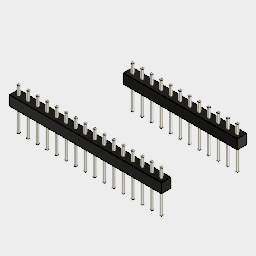
Standard Feather Pins (Autodesk Fusion 360 design; units mm, degrees)
Autodesk Fusion 360 part; units mm, degrees
note: some values were not read from the file. Chosen so that the rebuilt part matches the saved one: which bodies a step acts on.
sketch "pcb" plane through (0, 0, 0) normal (0, 0, 1) x (1, 0, 0)
  line L0 (0, 0) -> (51.2, 0)
  line L1 (51.2, 0) -> (51.2, 22.8)
  line L2 (51.2, 22.8) -> (0, 22.8)
  line L3 (0, 22.8) -> (0, 0)
  circle A0 centre (2.54, 2.54) radius 1.25
  circle A1 centre (2.54, 20.32) radius 1.25
  circle A2 centre (48.26, 20.32) radius 1.25
  circle A3 centre (48.26, 2.54) radius 1.25
  line L4 (0, 11.4) -> (51.2, 11.4) construction
  line L5 (25.6, 22.8) -> (25.6, 0) construction
  line L6 (0, 1.27) -> (51.2, 1.27) construction
  circle A4 centre (24.33, 1.27) radius 0.35
  circle A5 centre (21.79, 1.27) radius 0.35
  circle A6 centre (19.25, 1.27) radius 0.35
  circle A7 centre (16.71, 1.27) radius 0.35
  circle A8 centre (14.17, 1.27) radius 0.35
  circle A9 centre (11.63, 1.27) radius 0.35
  circle A10 centre (6.55, 1.27) radius 0.35
  circle A11 centre (26.87, 1.27) radius 0.35
  circle A12 centre (29.41, 1.27) radius 0.35
  circle A13 centre (31.95, 1.27) radius 0.35
  circle A14 centre (34.49, 1.27) radius 0.35
  circle A15 centre (39.57, 1.27) radius 0.35
  circle A16 centre (37.03, 1.27) radius 0.35
  circle A17 centre (42.11, 1.27) radius 0.35
  circle A18 centre (44.65, 1.27) radius 0.35
  circle A19 centre (44.65, 21.53) radius 0.35
  circle A20 centre (39.57, 21.53) radius 0.35
  circle A21 centre (34.49, 21.53) radius 0.35
  circle A22 centre (31.95, 21.53) radius 0.35
  circle A23 centre (29.41, 21.53) radius 0.35
  circle A24 centre (26.87, 21.53) radius 0.35
  circle A25 centre (42.11, 21.53) radius 0.35
  circle A26 centre (37.03, 21.53) radius 0.35
  circle A27 centre (24.33, 21.53) radius 0.35
  circle A28 centre (21.79, 21.53) radius 0.35
  circle A29 centre (19.25, 21.53) radius 0.35
  circle A30 centre (16.71, 21.53) radius 0.35
  line L7 (0, 2.54) -> (51.2, 2.54) construction
  circle A31 centre (9.09, 1.27) radius 0.35
  line L8 (45.92, 2.54) -> (5.28, 2.54)
  line L9 (5.28, 2.54) -> (5.28, 0)
  line L10 (5.28, 0) -> (45.92, 0)
  line L11 (45.92, 0) -> (45.92, 2.54)
  line L12 (45.92, 2.54) -> (5.28, 0) construction
  line L13 (5.28, 2.54) -> (45.92, 0) construction
  line L14 (45.92, 22.8) -> (15.44, 22.8)
  line L15 (15.44, 22.8) -> (15.44, 20.26)
  line L16 (15.44, 20.26) -> (45.92, 20.26)
  line L17 (45.92, 20.26) -> (45.92, 22.8)
  line L18 (45.92, 22.8) -> (15.44, 20.26) construction
  line L19 (15.44, 22.8) -> (45.92, 20.26) construction
  point P0 (25.6, 1.27)
  point P1 (30.68, 21.53)
  dimension "d1" = 51.2
  dimension "d2" = 22.8
  dimension "d3" = 2.5
  dimension "d4" = 2.54
  dimension "d5" = 2.54
  dimension "d6" = 2.5
  dimension "d7" = 2.54
  dimension "d8" = 20.32
  dimension "d9" = 2.5
  dimension "d10" = 48.26
  dimension "d11" = 20.32
  dimension "d12" = 2.5
  dimension "d13" = 2.54
  dimension "d14" = 48.26
  dimension "d40" = 1.27
  dimension "d41" = 0.7
  dimension "d42" = 1.27
  dimension "d43" = 0.7
  dimension "d44" = 0.7
  dimension "d45" = 0.7
  dimension "d46" = 0.7
  dimension "d47" = 2.54
  dimension "d48" = 2.54
  dimension "d49" = 2.54
  dimension "d50" = 2.54
  dimension "d51" = 0.7
  dimension "d53" = 0.7
  dimension "d55" = 2.54
  dimension "d58" = 0.7
  dimension "d59" = 0.7
  dimension "d60" = 0.7
  dimension "d61" = 0.7
  dimension "d62" = 2.54
  dimension "d63" = 2.54
  dimension "d64" = 2.54
  dimension "d65" = 1.27
  dimension "d68" = 0.7
  dimension "d74" = 0.7
  dimension "d75" = 2.54
  dimension "d76" = 2.54
  dimension "d77" = 0.7
  dimension "d78" = 0.7
  dimension "d79" = 2.54
  dimension "d80" = 2.54
  dimension "d95" = 1.27
  dimension "d133" = 0.7
  dimension "d134" = 2.54
  dimension "d135" = 2.54
  dimension "d165" = 2.54
  dimension "d166" = 40.64
  dimension "d167" = 30.48
  dimension "d168" = 2.54
  dimension "d169" = 1.27
  dimension "d170" = 1.27
  measures "d1" distance of L1.end L2.end
  measures "d2" distance of L0.end L1.end
  measures "d3" diameter of A0
  measures "d4" distance of L3 A0.centre
  measures "d5" distance of L0 A0.centre
  measures "d6" diameter of A1
  measures "d7" distance of L3 A1.centre
  measures "d8" distance of L0 A1.centre
  measures "d9" diameter of A2
  measures "d10" distance of L3 A2.centre
  measures "d11" distance of L0 A2.centre
  measures "d12" diameter of A3
  measures "d13" distance of L0 A3.centre
  measures "d14" distance of L3 A3.centre
  measures "d40" distance of L0 L6
  measures "d41" diameter of A4
  measures "d42" distance of L5 A4.centre
  measures "d43" diameter of A5
  measures "d44" diameter of A6
  measures "d45" diameter of A7
  measures "d46" diameter of A8
  measures "d47" distance of A4.centre A5.centre
  measures "d48" distance of A5.centre A6.centre
  measures "d49" distance of A6.centre A7.centre
  measures "d50" distance of A7.centre A8.centre
  measures "d51" diameter of A9
  measures "d53" diameter of A10
  measures "d55" distance of A8.centre A9.centre
  measures "d58" diameter of A11
  measures "d59" diameter of A12
  measures "d60" diameter of A13
  measures "d61" diameter of A14
  measures "d62" distance of A13.centre A14.centre
  measures "d63" distance of A12.centre A13.centre
  measures "d64" distance of A11.centre A12.centre
  measures "d65" distance of L5 A11.centre
  measures "d68" diameter of A15
  measures "d74" diameter of A16
  measures "d75" distance of A14.centre A16.centre
  measures "d76" distance of A15.centre A16.centre
  measures "d77" diameter of A17
  measures "d78" diameter of A18
  measures "d79" distance of A15.centre A17.centre
  measures "d80" distance of A17.centre A18.centre
  measures "d95" distance of L6 L7
  measures "d133" diameter of A31
  measures "d134" distance of A9.centre A31.centre
  measures "d135" distance of A10.centre A31.centre
  measures "d165" distance of L8.end L9.end
  measures "d166" distance of L9.end L10.end
  measures "d167" distance of L15.end L16.end
  measures "d168" distance of L14.end L15.end
  measures "d169" distance of L2 P1
  measures "d170" distance of A23.centre P1
extrude "Extrude3" add sketch "pcb" against normal blind 2.6 contours L0 L8 L9 L10 L11 | L2 L14 L15 L16 L17 | A4 | A5 | A6 | A7 | A8 | A9 | A10 | A11 | A12 | A13 | A14 | A15 | A16 | A17 | A18 | A19 | A20 | A21 | A22 | A23 | A24 | A25 | A26 | A27 | A28 | A29 | A30 | A31 makes body 1 at (35.76, 22.8, -0.8667) makes body 2 at (32.3733, 0, -1.7333) in component "Header Strip"
extrude "Extrude2" add sketch "pcb" along normal blind 2.6 and the other way blind 9.05 separate body contours A4 | A5 | A6 | A7 | A8 | A9 | A10 | A11 | A12 | A13 | A14 | A15 | A16 | A17 | A18 | A19 | A20 | A21 | A22 | A23 | A24 | A25 | A26 | A27 | A28 | A29 | A30 | A31 makes body 3 at (11.6213, 1.6199, -6.0333) makes body 4 at (21.6303, 0.9585, -6.0333) makes body 5 at (32.1399, 1.564, -6.0333) makes body 6 at (42.2999, 1.564, -6.0333) makes body 7 at (39.3801, 21.236, -6.0333) makes body 8 at (29.554, 21.849, -6.0333) makes body 9 at (19.394, 21.849, -6.0333) makes body 10 at (21.934, 21.849, -6.0333) makes body 11 at (32.1399, 21.236, -3.0167) makes body 12 at (41.9201, 21.236, -6.0333) makes body 13 at (39.7599, 1.564, -6.0333) makes body 14 at (29.2503, 0.9585, -6.0333) makes body 15 at (19.394, 1.589, -6.0333) makes body 16 at (9.0813, 1.6199, -6.0333) makes body 17 at (14.1613, 1.6199, -6.0333) makes body 18 at (24.1703, 0.9585, -6.0333) makes body 19 at (34.6799, 1.564, -6.0333) makes body 20 at (44.8399, 1.564, -6.0333) makes body 21 at (36.8401, 21.236, -6.0333) makes body 22 at (27.014, 21.849, -6.0333) makes body 23 at (16.854, 21.849, -6.0333) makes body 24 at (24.474, 21.849, -6.0333) makes body 25 at (34.3001, 21.236, -6.0333) makes body 26 at (44.4601, 21.236, -6.0333) makes body 27 at (37.2199, 1.564, -6.0333) makes body 28 at (26.7103, 0.9585, -6.0333) makes body 29 at (16.854, 1.589, -6.0333) makes body 30 at (6.8983, 1.2352, -6.0333) in component "Pins"
fillet "Fillet3" radius 0.3 56 edges at (11.3037, 1.3966, -9.05) (11.3037, 1.1434, 2.6) (21.4637, 1.3966, -9.05) (21.4637, 1.1434, 2.6) (31.6237, 1.3966, -9.05) (31.6237, 1.1434, 2.6) (41.7837, 1.1434, 2.6) (41.7837, 1.3966, -9.05) (39.2437, 21.6566, -9.05) (39.2437, 21.4034, 2.6) (29.0837, 21.6566, -9.05) (29.0837, 21.4034, 2.6) (18.9237, 21.6566, -9.05) (18.9237, 21.4034, 2.6) (21.4637, 21.6566, -9.05) (21.4637, 21.4034, 2.6) (31.6237, 21.6566, -9.05) (31.6237, 21.4034, 2.6) (41.7837, 21.6566, -9.05) (41.7837, 21.4034, 2.6) (39.2437, 1.1434, 2.6) (39.2437, 1.3966, -9.05) (29.0837, 1.3966, -9.05) (29.0837, 1.1434, 2.6) (18.9237, 1.1434, 2.6) (18.9237, 1.3966, -9.05) (8.7637, 1.1434, 2.6) (8.7637, 1.3966, -9.05) (13.8437, 1.3966, -9.05) (13.8437, 1.1434, 2.6) (24.0037, 1.1434, 2.6) (24.0037, 1.3966, -9.05) (34.1637, 1.1434, 2.6) (34.1637, 1.3966, -9.05) (44.3237, 1.1434, 2.6) (44.3237, 1.3966, -9.05) (36.7037, 21.4034, 2.6) (36.7037, 21.6566, -9.05) (26.5437, 21.6566, -9.05) (26.5437, 21.4034, 2.6) (16.3837, 21.6566, -9.05) (16.3837, 21.4034, 2.6) (24.0037, 21.6566, -9.05) (24.0037, 21.4034, 2.6) (34.1637, 21.6566, -9.05) (34.1637, 21.4034, 2.6) (44.3237, 21.4034, 2.6) (44.3237, 21.6566, -9.05) (36.7037, 1.3966, -9.05) (36.7037, 1.1434, 2.6) (26.5437, 1.3966, -9.05) (26.5437, 1.1434, 2.6) (16.3837, 1.3966, -9.05) (16.3837, 1.1434, 2.6) (6.2237, 1.3966, -9.05) (6.2237, 1.1434, 2.6) on bodies 3 4 5 6 7 8 9 10 11 12 13 14 15 16 17 18 19 20 21 22 23 24 25 26 27 28 29 30 in component "Pins"
component "Header Strip" placed x (1, 0, 0) y (0, 1, 0) z (0, 0, 1) at (0, 0, 0)
component "Pins" placed x (1, 0, 0) y (0, 1, 0) z (0, 0, 1) at (0, 0, 0)
equation "PinDia = 0.7 mm"
equation "HoleSpace = 0.1 in"
equation "Hole2Edge = 0.05 in"
equation "d40 = Hole2Edge"
equation "d41 = PinDia"
equation "d42 = HoleSpace / 2"
equation "d43 = PinDia"
equation "d44 = PinDia"
equation "d45 = PinDia"
equation "d46 = PinDia"
equation "d47 = HoleSpace"
equation "d48 = HoleSpace"
equation "d49 = HoleSpace"
equation "d50 = HoleSpace"
equation "d51 = PinDia"
equation "d53 = PinDia"
equation "d55 = HoleSpace"
equation "d58 = PinDia"
equation "d59 = PinDia"
equation "d60 = PinDia"
equation "d61 = PinDia"
equation "d62 = HoleSpace"
equation "d63 = HoleSpace"
equation "d64 = HoleSpace"
equation "d65 = HoleSpace / 2"
equation "d68 = PinDia"
equation "d74 = PinDia"
equation "d75 = HoleSpace"
equation "d76 = HoleSpace"
equation "d77 = PinDia"
equation "d78 = PinDia"
equation "d79 = HoleSpace"
equation "d80 = HoleSpace"
equation "d95 = HoleSpace / 2"
equation "d133 = PinDia"
equation "d134 = HoleSpace"
equation "d135 = HoleSpace"
equation "d175 = 6.25 mm + 2.8 mm"
